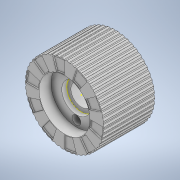
# Autodesk Inventor part: runner
Saved by Autodesk Inventor 2022 (Build 260153000, 153)
## iProperties
Created: 2023-12-11
Part Number: runner
Material: Generisch
Document SubType Name: Modeling
Designer: Marc Panse
Density: 1 g/cm^3
Appearance: Vorgabe
Author: Marc Panse
## iProperties of the stored document runner_3D-Druck.ipt
Created: 2023-12-11
Part Number: runner_3D-Druck
Material: Generisch
Document SubType Name: Modeling
Designer: Marc Panse
Density: 1 g/cm^3
Appearance: Vorgabe
Author: Marc Panse
Autodesk Inventor part; units mm, degrees
ref_plane "YZ Plane" through (0, 0, 0) normal (1, 0, 0) x (0, 1, 0)
ref_plane "XZ Plane" through (0, 0, 0) normal (0, 1, 0) x (-1, 0, 0)
ref_plane "XY Plane" through (0, 0, 0) normal (0, 0, 1) x (1, 0, 0)
sketch "Skizze1" plane through (0, 0, 0) normal (0, 0, 1) x (1, 0, 0)
  circle A0 centre (0, 0) radius 24
  circle A1 centre (0, 0) radius 28.2
  dimension "d0" = 48
  dimension "d1" = 56.4
  constraints: 2 centre point, 2 coincident
  measures "d0" diameter of A0
  measures "d1" diameter of A1
extrude "Extrusion1" add sketch "Skizze1" along normal blind 14
sketch "Skizze2" plane through (0, 0, 0) normal (0, 0, -1) x (-1, 0, 0)
  circle A0 centre (0, 0) radius 24.95
  dimension "d4" = 49.9
  constraints: 1 centre point, 1 coincident
  measures "d4" diameter of A0
extrude "Extrusion2" cut sketch "Skizze2" against normal blind 0.9
sketch "Skizze3" plane through (0, 0, 14) normal (0, 0, 1) x (1, 0, 0)
  circle A0 centre (0, 0) radius 28.2 projected
  circle A1 centre (0, 0) radius 24 projected
  circle A2 centre (0, 0) radius 11.5
  dimension "d7" = 23
  constraints: 1 centre point, 1 coincident
  measures "d7" diameter of A2
extrude "Extrusion3" add sketch "Skizze3" along normal blind 7.4 contours A0 | A1
sketch "Skizze4" plane through (0, 0, 21.4) normal (0, 0, 1) x (1, 0, 0)
  circle A0 centre (0, 0) radius 10.5
  circle A1 centre (0, 0) radius 28.2 projected
  circle A2 centre (0, 0) radius 11.5 projected
  dimension "d10" = 21
  constraints: 1 centre point, 1 coincident
  measures "d10" diameter of A0
extrude "Extrusion4" add sketch "Skizze4" against normal blind 5 contours A2
sketch "Skizze5" plane through (0, 0, 21.4) normal (0, 0, 1) x (1, 0, 0)
  circle A0 centre (0, 0) radius 29.0057
  circle A1 centre (0, 0) radius 10.8
  circle A2 centre (0, 0) radius 18
  circle A3 centre (0, 0) radius 10.5 projected
  circle A4 centre (0, 0) radius 28.2 projected
  dimension "d13" = 36
  constraints: 3 centre point, 3 coincident
  measures "d13" diameter of A2
extrude "Extrusion5" add sketch "Skizze5" along normal blind 7 contours A4
sketch "Skizze6" plane through (0, 0, 14) normal (0, 0, -1) x (-1, 0, 0)
  circle A0 centre (0, 0) radius 11.5 projected
  circle A1 centre (0, 0) radius 24 projected
extrude "Extrusion6" add sketch "Skizze6" along normal blind 8
sketch "Skizze7" plane through (0, 0, 0) normal (0, 0, -1) x (-1, 0, 0)
  point P0 (0, 0)
sketch "Skizze8" plane through (0, 0, 0) normal (0, 0, -1) x (-1, 0, 0)
  circle A0 centre (0, 0) radius 24.95 projected
  circle A1 centre (0, 0) radius 28.2 projected
extrude "Extrusion7" add sketch "Skizze8" along normal blind 8
sketch "Skizze9" plane through (0, 0, 0.9) normal (0, 0, -1) x (-1, 0, 0)
  circle A0 centre (0, 0) radius 24 projected
  circle A1 centre (0, 0) radius 24.95 projected
extrude "Extrusion8" add sketch "Skizze9" along normal blind 8
sketch "Skizze10" plane through (0, 0, 21.4) normal (0, 0, 1) x (1, 0, 0)
  circle A0 centre (0, 0) radius 13.758
  circle A1 centre (0, -13.758) radius 3.05
  dimension "d22" = 27.516
  dimension "d23" = 6.1
  constraints: 1 centre point, 1 coincident, 1 vertical alignment, 2 other
  measures "d23" diameter of A1
extrude "Extrusion9" cut sketch "Skizze10" against normal blind 14 contours A1 A0 | A0 A1 picked at (0, -12.7162) picked at (-0.0564, -14.748)
sketch "Skizze11" plane through (0, 0, -8) normal (0, 0, -1) x (-1, 0, 0)
  circle A0 centre (0, 0) radius 28.2 projected
  circle A1 centre (0, -28.2) radius 0.6087
  constraints: 1 centre point, 1 vertical alignment, 1 other
extrude "Extrusion10" cut sketch "Skizze11" against normal blind 57 contours A1 A0 | A0 A1 picked at (-0.0243, -27.9981) picked at (0.0235, -28.4011)
fillet "Rundung1" radius 2 4 edges at (-0.6086, -28.1934, -4) (-0.6086, -28.1934, 14.2) (0.6086, -28.1934, -4) (0.6086, -28.1934, 14.2)
pattern_circular "Runde Anordnung1" count 50 over 360 about axis through (0, 0, -10) along (0, 0, 1) of "Extrusion10", "Rundung1"
sketch "Skizze13" plane through (0, 0, 28.4) normal (0, 0, 1) x (1, 0, 0)
  circle A0 centre (0, 0) radius 18.165
  dimension "d35" = 36.33
  constraints: 1 centre point, 1 coincident
  measures "d35" diameter of A0
extrude "Extrusion12" cut sketch "Skizze13" against normal up to surface (7 mm away)
sketch "Skizze14" plane through (0, 0, 21.4) normal (0, 0, 1) x (1, 0, 0)
  circle A0 centre (0, -13.758) radius 3.05 projected
  circle A1 centre (0, -13.758) radius 3.15
  point P0 (0, 0)
  dimension "d38" = 6.3
  constraints: 1 centre point, 1 coincident
  measures "d38" diameter of A1
extrude "Extrusion13" cut sketch "Skizze14" against normal up to surface (14 mm away) contours A0 | A1
sketch "Skizze15" plane through (0, 0, 21.4) normal (0, 0, 1) x (1, 0, 0)
  circle A0 centre (0, -13.758) radius 3.15 projected
  circle A1 centre (0, 0) radius 18.165 projected
  circle A2 centre (0, 0) radius 10.5 projected
extrude "Extrusion14" cut sketch "Skizze15" against normal blind 1.5
sketch "Skizze16" plane through (0, 0, -8) normal (0, 0, -1) x (-1, 0, 0)
  circle A0 centre (0, 0) radius 25.1
  dimension "d43" = 50.2
  constraints: 1 centre point, 1 coincident
  measures "d43" diameter of A0
extrude "Extrusion15" cut sketch "Skizze16" against normal up to surface (0.9 mm away)
sketch "Skizze17" plane through (0, 0, 6) normal (0, 0, -1) x (-1, 0, 0)
  circle A0 centre (0, 0) radius 24 projected
  circle A1 centre (0, 0) radius 11.5 projected
extrude "Extrusion16" cut sketch "Skizze17" against normal blind 0.5
sketch "Skizze18" plane through (0, 0, -7.1) normal (0, 0, -1) x (-1, 0, 0)
  circle A0 centre (0, 0) radius 25.1 projected
  circle A1 centre (0, 0) radius 24 projected
extrude "Extrusion17" cut sketch "Skizze18" against normal blind 0.5
sketch "Skizze19" plane through (0, 0, -8) normal (0, 0, -1) x (-1, 0, 0)
  circle A0 centre (0, 0) radius 24.5
  dimension "d50" = 49
  constraints: 1 centre point, 1 coincident
  measures "d50" diameter of A0
extrude "Extrusion18" cut sketch "Skizze19" against normal up to surface (14.5 mm away)
sketch "Skizze20" plane through (0, 0, 6.5) normal (0, 0, -1) x (-1, 0, 0)
  circle A0 centre (0, 0) radius 12
  dimension "d53" = 24
  constraints: 1 centre point, 1 coincident
  measures "d53" diameter of A0
extrude "Extrusion19" cut sketch "Skizze20" against normal blind 3
sketch "Skizze21" plane through (0, 0, 9.5) normal (0, 0, -1) x (-1, 0, 0)
  circle A0 centre (0, 0) radius 10.5
  circle A1 centre (0, 0) radius 7.5
  dimension "d56" = 15
  constraints: 2 centre point, 2 coincident
  measures "d56" diameter of A1
extrude "Extrusion20" add sketch "Skizze21" against normal up to surface (6.9 mm away)
sketch "Skizze22" plane through (0, 0, 9.5) normal (0, 0, -1) x (-1, 0, 0)
  circle A0 centre (0, 0) radius 10.5 projected
  arc A1 (2.0004, -11.3247) -> (-2.0004, -11.3247) centre (0, -13.758) ccw projected
  arc A2 (2.0004, -11.3247) -> (-2.0004, -11.3247) centre (0, 0) ccw projected
sketch "Skizze23" plane through (0, 0, 9.5) normal (0, 0, -1) x (-1, 0, 0)
  arc A0 (-2.0004, -11.3247) -> (-2.4284, -11.7517) centre (0, -13.758) ccw projected
  arc A1 (2.0004, -11.3247) -> (-2.0004, -11.3247) centre (0, 0) ccw projected
  arc A2 (2.4284, -11.7517) -> (2.0004, -11.3247) centre (0, -13.758) ccw projected
  arc A3 (2.4284, -11.7517) -> (-2.4284, -11.7517) centre (0, 0) ccw projected
extrude "Extrusion21" add sketch "Skizze23" along normal blind 1
sketch "Skizze24" plane through (0, 0, 16.4) normal (0, 0, -1) x (-1, 0, 0)
  circle A0 centre (0, 0) radius 10.5 projected
  arc A1 (2.0004, -11.3247) -> (-2.0004, -11.3247) centre (0, -13.758) ccw projected
  arc A2 (2.0004, -11.3247) -> (-2.0004, -11.3247) centre (0, 0) ccw projected
extrude "Extrusion22" add sketch "Skizze22" against normal up to surface (6.9 mm away)
sketch "Skizze25" plane through (0, 0, 28.4) normal (0, 0, 1) x (1, 0, 0)
  arc A0 (-0.3765, 27.7217) -> (0.3765, 27.7217) centre (0, 28.2) ccw projected
  circle A1 centre (0, 0) radius 27.7243
  circle A2 centre (0, 0) radius 18.165 projected
  line L0 (0, -18.165) -> (0, -27.7243)
  line L1 (-5.6133, -17.2759) -> (-8.5673, -26.3674)
  line L2 (-10.6771, -14.6958) -> (-16.2959, -22.4294)
  line L3 (-14.6958, -10.6771) -> (-22.4294, -16.2959)
  line L4 (-17.2759, -5.6133) -> (-26.3674, -8.5673)
  line L5 (-18.165, 0) -> (-27.7243, 0)
  line L6 (-17.2759, 5.6133) -> (-26.3674, 8.5673)
  line L7 (-14.6958, 10.6771) -> (-22.4294, 16.2959)
  line L8 (-10.6771, 14.6958) -> (-16.2959, 22.4294)
  line L9 (-5.6133, 17.2759) -> (-8.5673, 26.3674)
  line L10 (0, 18.165) -> (0, 27.7243)
  line L11 (5.6133, 17.2759) -> (8.5673, 26.3674)
  line L12 (10.6771, 14.6958) -> (16.2959, 22.4294)
  line L13 (14.6958, 10.6771) -> (22.4294, 16.2959)
  line L14 (17.2759, 5.6133) -> (26.3674, 8.5673)
  line L15 (18.165, 0) -> (27.7243, 0)
  line L16 (17.2759, -5.6133) -> (26.3674, -8.5673)
  line L17 (14.6958, -10.6771) -> (22.4294, -16.2959)
  line L18 (10.6771, -14.6958) -> (16.2959, -22.4294)
  line L19 (5.6133, -17.2759) -> (8.5673, -26.3674)
  circle A3 centre (0, 0) radius 18.665
  circle A4 centre (0, 0) radius 27.3453
  point P0 (-16.0731, 22.1228)
  point P1 (-22.1228, 16.0731)
  point P2 (-15.1003, 10.971)
  point P3 (-10.971, 15.1003)
  point P4 (-26.0069, 8.4501)
  point P5 (-27.3453, 0)
  point P6 (-18.665, 0)
  point P7 (-17.7515, 5.7678)
  point P8 (-26.0069, -8.4501)
  point P9 (-22.1228, -16.0731)
  point P10 (-15.1003, -10.971)
  point P11 (-17.7515, -5.7678)
  point P12 (-16.0731, -22.1228)
  point P13 (-8.4501, -26.0069)
  point P14 (-5.7678, -17.7515)
  point P15 (-10.971, -15.1003)
  point P16 (0, -27.3453)
  point P17 (8.4501, -26.0069)
  point P18 (5.7678, -17.7515)
  point P19 (0, -18.665)
  point P20 (16.0731, -22.1228)
  point P21 (22.1228, -16.0731)
  point P22 (15.1003, -10.971)
  point P23 (10.971, -15.1003)
  point P24 (26.0069, -8.4501)
  point P25 (27.3453, 0)
  point P26 (18.665, 0)
  point P27 (17.7515, -5.7678)
  point P28 (26.0069, 8.4501)
  point P29 (22.1228, 16.0731)
  point P30 (15.1003, 10.971)
  point P31 (17.7515, 5.7678)
  point P32 (16.0731, 22.1228)
  point P33 (8.4501, 26.0069)
  point P34 (5.7678, 17.7515)
  point P35 (10.971, 15.1003)
  point P36 (0, 27.3453)
  point P37 (-8.4501, 26.0069)
  point P38 (-5.7678, 17.7515)
  point P39 (0, 18.665)
  dimension "d65" = 360
  dimension "d67" = 37.33
  constraints: 40 end point, 5 coincident, 3 centre point, 2 point on circle, 1 vertical, 1 vertical alignment, 80 other
  measures "d67" diameter of A3
extrude "Extrusion23" cut sketch "Skizze25" against normal blind 1 contours L10 A3 L9 A4 | A4 L12 A3 L11 | L8 A3 L7 A4 | A4 L14 A3 L13 | L6 A3 L5 A4 | A4 L16 A3 L15 | L4 A3 L3 A4 | A4 L18 A3 L17 | L2 A3 L1 A4 | A4 L0 A3 L19
